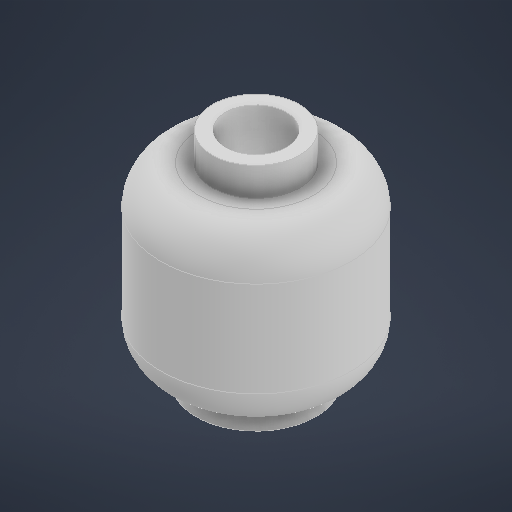
# Autodesk Inventor part: Lego head
Saved by Autodesk Inventor 2027.1 (Build 311270010, 270A)
## iProperties
Created: 2020-11-13
Part Number: Lego head
Material: Generic
Document SubType Name: Modeling
Designer: 164344
Density: 1 g/cm^3
Appearance: Default
Author: 164344
Autodesk Inventor part; units mm, degrees
ref_plane "YZ Plane" through (0, 0, 0) normal (1, 0, 0) x (0, 1, 0)
ref_plane "XZ Plane" through (0, 0, 0) normal (0, 1, 0) x (-1, 0, 0)
ref_plane "XY Plane" through (0, 0, 0) normal (0, 0, 1) x (1, 0, 0)
sketch "Sketch1" plane through (0, 0, 0) normal (0, 0, 1) x (1, 0, 0)
  line L0 (0, 0) -> (0, 11.5)
  line L1 (0, 0) -> (-3.15, 0)
  line L2 (-3.15, 0) -> (-3.15, 1)
  arc A0 (-5, 3) -> (-3.15, 1) centre (-2.9939, 3) ccw
  line L3 (-5, 3) -> (-5, 8)
  arc A1 (-3, 10) -> (-5, 8) centre (-3, 8) ccw
  line L4 (-3, 10) -> (-2.3, 10)
  line L5 (-2.3, 10) -> (-2.3, 11.5)
  line L6 (-2.3, 11.5) -> (0, 11.5)
  dimension "d0" = 11.5
  dimension "d1" = 3.15
  dimension "d2" = 1
  dimension "d3" = 5
  dimension "d4" = 5
  dimension "d5" = 2.3
  dimension "d7" = 2
  dimension "d8" = 2
  dimension "d9" = 2
  constraints: 14 end point, 4 point on circle, 3 horizontal, 3 vertical, 2 centre point, 2 tangent, 1 perpendicular
  measures "d0" distance of L0.start L0.end
  measures "d1" distance of L0.start L1.end
  measures "d2" distance of L1.end L2.end
  measures "d3" distance of L3.start L3.end
  measures "d4" distance between parallel lines of L0 L3
  measures "d5" distance between parallel lines of L0 L5
  measures "d7" horizontal distance of L3.end L4.start
  measures "d8" horizontal distance of L4.start L3.end
  measures "d9" vertical distance of L3.start L2.end
revolve "Revolution1" add sketch "Sketch1" angle 360 about axis through (0, 0, 0) along (0, 1, 0)
sketch "Sketch2" plane through (0, 0, 0) normal (0, -1, 0) x (1, 0, 0)
  circle A0 centre (0, 0) radius 2.5975
  dimension "d11" = 5.195
  constraints: 1 centre point, 1 coincident
  measures "d11" diameter of A0
extrude "Extrusion1" cut sketch "Sketch2" against normal blind 8.6
sketch "Sketch3" plane through (0, 11.5, 0) normal (0, 1, 0) x (1, 0, 0)
  circle A0 centre (0, 0) radius 2.3 projected
  circle A1 centre (0, 0) radius 1.6
  dimension "d14" = 0.7
  constraints: 1 centre point
  measures "d14" radial gap between concentric circles of A0 A1
extrude "Extrusion2" cut sketch "Sketch3" against normal blind 2.2 contours A1
sketch "Sketch4" plane through (0, 9.3, 0) normal (0, 1, 0) x (1, 0, 0)
  circle A0 centre (0, 0) radius 0.4 construction
  circle A1 centre (0, 0) radius 1.6 projected
  line L0 (-1.5639, 0.338) -> (-0.2139, 0.338)
  line L1 (-0.2139, 0.338) -> (0.4734, 1.5284)
  arc A2 (0.4734, 1.5284) -> (-1.5639, 0.338) centre (0, 0) ccw
  dimension "d17" = 0.8
  dimension "d18" = 1.35
  dimension "d19" = 120
  constraints: 4 end point, 4 point on circle, 1 centre point, 1 coincident, 1 concentric, 1 horizontal, 3 other
  measures "d18" distance of L0.start L0.end
  measures "d19" angle of L1 L0
extrude "Extrusion3" cut sketch "Sketch4" against normal blind 4 contours L1 L0 A1 picked at (0.1203, 1.1544)
pattern_circular "Circular Pattern1" count 3 over 360 about axis through (0, 11.5, 0) along (0, -1, 0) of "Extrusion3"
sketch "Sketch5" plane through (0, 9.3, 0) normal (0, 1, 0) x (1, 0, 0)
  circle A0 centre (0, 0) radius 0.25
  dimension "d25" = 0.5
  constraints: 1 centre point, 1 coincident
  measures "d25" diameter of A0
extrude "Extrusion4" cut sketch "Sketch5" against normal blind 0.2
body "Solid1"
